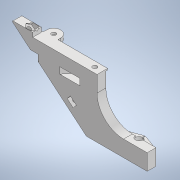
# Autodesk Inventor part: sciana
Saved by Autodesk Inventor 2022 (Build 260153000, 153)
## iProperties
Created: 2022-12-26
Part Number: sciana
Material: Generic
Document SubType Name: Modeling
Designer: Kamil
Density: 1 g/cm^3
Appearance: Default
Author: Kamil
Autodesk Inventor part; units mm, degrees
ref_plane "YZ Plane" through (0, 0, 0) normal (1, 0, 0) x (0, 1, 0)
ref_plane "XZ Plane" through (0, 0, 0) normal (0, 1, 0) x (-1, 0, 0)
ref_plane "XY Plane" through (0, 0, 0) normal (0, 0, 1) x (1, 0, 0)
sketch "Sketch1" plane through (0, 0, 0) normal (0, 0, 1) x (1, 0, 0)
  line L0 (7.1699, 8.5) -> (10.7451, 5.5) projected
  line L1 (65.8, 5.5) -> (10.7451, 5.5) projected
  line L2 (65.8, 5.5) -> (65.8, 8.5) projected
  line L3 (65.8, 8.5) -> (7.1699, 8.5) projected
  line L4 (10.7451, 5.5) -> (39.9536, -19.0089)
  circle A0 centre (83.9, -5.5) radius 16.1 projected
  line L5 (83.9, 8.5) -> (65.8, 8.5) projected
  line L6 (65.8, 5.5) -> (65.8, -20.8049)
  line L7 (65.8, -20.8049) -> (42.0941, -20.8049)
  line L8 (42.0941, -20.8049) -> (39.9536, -19.0089)
  circle A1 centre (83.9, -5.5) radius 18.1
  line L9 (83.9, -23.6) -> (100, -23.6)
  line L10 (100, -23.6) -> (100, -27.6)
  line L11 (100, -27.6) -> (50.1922, -27.6)
  line L12 (50.1922, -27.6) -> (42.0941, -20.8049)
  point P0 (0, 0)
  point P1 (65.8, -5.5)
  dimension "d0" = 4
  constraints: 16 end point, 3 perpendicular, 2 collinear, 2 horizontal, 2 vertical, 1 coincident, 3 other
  measures "d0" distance of L9.end L10.end
extrude "Extrusion1" add sketch "Sketch1" against normal blind 6 contours L1 L6 L7 L8 L4 | A1 L9 L10 L11 L12 L7 L6
sketch "Sketch2" plane through (10.7451, 5.5, 0) normal (0, 1, 0) x (1, 0, 0)
  line L0 (21.4448, 9) -> (21.4448, 14.7444) projected
  line L1 (85.3549, 52.5) -> (85.3549, 47.5) projected
  line L2 (85.3549, 47.5) -> (41.1549, 47.5) projected
  line L3 (41.1549, 47.5) -> (41.1549, 32) projected
  line L4 (41.1549, 32) -> (52.3217, 32) projected
  line L5 (52.3217, 32) -> (52.3217, 9) projected
  line L6 (52.3217, 9) -> (21.4448, 9) projected
  line L7 (21.4448, 9) -> (21.4448, 14.7444) projected
  line L8 (21.4448, 14.7444) -> (11.2254, 14.7444) projected
  line L9 (11.2254, 14.7444) -> (11.2254, 9) projected
  line L10 (11.2254, 9) -> (3.1975, 9) projected
  line L11 (3.1975, 9) -> (3.1975, 22) projected
  line L12 (3.1975, 22) -> (11.2254, 22) projected
  line L13 (11.2254, 22) -> (11.2254, 78) projected
  line L14 (11.2254, 78) -> (3.1975, 78) projected
  line L15 (3.1975, 78) -> (3.1975, 91) projected
  line L16 (3.1975, 91) -> (11.2254, 91) projected
  line L17 (11.2254, 91) -> (11.2254, 85.2556) projected
  line L18 (11.2254, 85.2556) -> (21.4448, 85.2556) projected
  line L19 (21.4448, 85.2556) -> (21.4448, 91) projected
  line L20 (21.4448, 91) -> (52.3217, 91) projected
  line L21 (52.3217, 91) -> (52.3217, 68) projected
  line L22 (52.3217, 68) -> (41.1549, 68) projected
  line L23 (41.1549, 68) -> (41.1549, 52.5) projected
  line L24 (41.1549, 52.5) -> (85.3549, 52.5) projected
  line L25 (22.6158, 64.3503) -> (20.3041, 53.9031) projected
  line L26 (20.3041, 53.9031) -> (21.8663, 53.5574) projected
  line L27 (21.8663, 53.5574) -> (24.178, 64.0047) projected
  line L28 (24.178, 64.0047) -> (22.6158, 64.3503) projected
  line L29 (20.2927, 51.2105) -> (22.6127, 40.765) projected
  line L30 (22.6127, 40.765) -> (24.1746, 41.112) projected
  line L31 (24.1746, 41.112) -> (21.8546, 51.5574) projected
  line L32 (21.8546, 51.5574) -> (20.2927, 51.2105) projected
  line L33 (25.3403, 18.5643) -> (24.1979, 17.4441) projected
  line L34 (24.1979, 17.4441) -> (31.6895, 9.8042) projected
  line L35 (31.6895, 9.8042) -> (32.8319, 10.9245) projected
  line L36 (32.8319, 10.9245) -> (25.3403, 18.5643) projected
  line L37 (37.3906, 88.6369) -> (36.265, 89.7739) projected
  line L38 (36.265, 89.7739) -> (28.6611, 82.2458) projected
  line L39 (28.6611, 82.2458) -> (29.7868, 81.1088) projected
  line L40 (29.7868, 81.1088) -> (37.3906, 88.6369) projected
  line L41 (37.3228, 15.3834) -> (36.9774, 13.8212) projected
  line L42 (36.9774, 13.8212) -> (47.4252, 11.5115) projected
  line L43 (47.4252, 11.5115) -> (47.7705, 13.0737) projected
  line L44 (47.7705, 13.0737) -> (37.3228, 15.3834) projected
  line L45 (51.9234, 89.2388) -> (51.5762, 90.8006) projected
  line L46 (51.5762, 90.8006) -> (41.1312, 88.4785) projected
  line L47 (41.1312, 88.4785) -> (41.4784, 86.9167) projected
  line L48 (41.4784, 86.9167) -> (51.9234, 89.2388) projected
  line L49 (39.447, 6) -> (0, 6) projected
  line L50 (0, 6) -> (55.0549, 6) projected
  line L51 (55.0549, 6) -> (73.1549, 6) projected
  line L52 (73.1549, 6) -> (89.2549, 6) projected
  line L53 (89.2549, 6) -> (39.447, 6) projected
  line L54 (16.3351, 14.7444) -> (16.3351, 5.7961)
  line L55 (39.447, 6) -> (0, 6) projected
  line L56 (16.3351, 6) -> (16.3351, 9.2)
  line L57 (14.4876, 6) -> (12.6401, 9.2)
  line L58 (12.6401, 9.2) -> (14.4876, 12.4)
  line L59 (14.4876, 12.4) -> (18.1826, 12.4)
  line L60 (18.1826, 12.4) -> (20.0302, 9.2)
  line L61 (20.0302, 9.2) -> (18.1826, 6)
  line L62 (18.1826, 6) -> (14.4876, 6)
  circle A0 centre (16.3351, 9.2) radius 4.75
  line L63 (11.5851, 9.2) -> (11.5851, 6)
  line L64 (21.0851, 9.2) -> (21.0851, 6)
  point P0 (-10.7451, 0)
  point P1 (11.5851, 6)
  point P2 (21.0851, 6)
  dimension "d3" = 3.2
  dimension "d4" = 9.5
  constraints: 20 end point, 5 point on line, 2 coincident, 2 midpoint, 2 perpendicular, 2 point on circle, 1 centre point, 1 tangent, 1 vertical, 13 other
  measures "d3" distance of L56.start L56.end
  measures "d4" diameter of A0
extrude "Extrusion2" add sketch "Sketch2" against normal blind 3 contours L61 L60 L59 L54 A0 L49 | A0 L64 L49 | L49 A0 L54 L59 L58 L57 | L49 L63 A0
sketch "Sketch3" plane through (10.7451, 5.5, 0) normal (0, 1, 0) x (1, 0, 0)
  line L0 (11.5851, 6) -> (14.4876, 6) projected
  line L1 (11.5851, 6) -> (11.5851, 9.2) projected
  arc A0 (21.0851, 9.2) -> (11.5851, 9.2) centre (16.3351, 9.2) ccw projected
  line L2 (21.0851, 9.2) -> (21.0851, 6) projected
  line L3 (18.1826, 6) -> (21.0851, 6) projected
  line L4 (18.1826, 6) -> (20.0302, 9.2) projected
  line L5 (20.0302, 9.2) -> (18.1826, 12.4) projected
  line L6 (18.1826, 12.4) -> (14.4876, 12.4) projected
  line L7 (14.4876, 12.4) -> (12.6401, 9.2) projected
  line L8 (12.6401, 9.2) -> (14.4876, 6) projected
  circle A1 centre (16.3351, 9.2) radius 1.5
  line L9 (14.4876, 6) -> (18.1826, 6) projected
  point P0 (-10.7451, 0)
  dimension "d7" = 3
  constraints: 1 centre point, 1 coincident
  measures "d7" diameter of A1
extrude "Extrusion3" add sketch "Sketch3" against normal blind 1.5 contours L8 L7 L6 L5 L4 L9
fillet "Fillet1" radius 2 4 edges at (31.8302, 4, -6) (22.3302, 4, -6) (30.379, 2.5, -6) (23.7815, 2.5, -6)
sketch "Sketch4" plane through (10.7451, 5.5, 0) normal (0, 1, 0) x (1, 0, 0)
  circle A0 centre (64.1549, 42.5) radius 1.75 projected
  circle A1 centre (64.1549, 57.5) radius 1.75 projected
  circle A2 centre (46.1549, 42.5) radius 1.5 projected
  circle A3 centre (46.1549, 57.5) radius 1.5 projected
  line L0 (-3.5753, 100) -> (-3.5753, 0) projected
  line L1 (55.0549, 0) -> (-3.5753, 0) projected
  line L2 (55.0549, 35) -> (55.0549, 0) projected
  line L3 (73.1549, 35) -> (55.0549, 35) projected
  line L4 (73.1549, 35) -> (73.1549, 65) projected
  line L5 (55.0549, 65) -> (73.1549, 65) projected
  line L6 (55.0549, 100) -> (55.0549, 65) projected
  line L7 (-3.5753, 100) -> (55.0549, 100) projected
  line L8 (23.0851, 6) -> (55.0549, 6) projected
  line L9 (55.0549, 0) -> (53.0549, 0)
  line L10 (53.0549, 0) -> (53.0549, 9.1684)
  line L11 (53.0549, 9.1684) -> (55.0549, 9.1684)
  line L12 (55.0549, 9.1684) -> (55.0549, 0)
  line L13 (53.0549, 0) -> (46.6549, 0)
  line L14 (46.6549, 0) -> (46.6549, 7.4)
  line L15 (46.6549, 7.4) -> (53.0549, 7.4)
  line L16 (53.0549, 7.4) -> (53.0549, 0)
  line L17 (46.6549, 3.7) -> (53.0549, 3.7)
  line L18 (46.6549, 5.5475) -> (49.8549, 7.395)
  line L19 (49.8549, 7.395) -> (53.0549, 5.5475)
  line L20 (53.0549, 5.5475) -> (53.0549, 1.8525)
  line L21 (53.0549, 1.8525) -> (49.8549, 0.005)
  line L22 (49.8549, 0.005) -> (46.6549, 1.8525)
  line L23 (46.6549, 1.8525) -> (46.6549, 5.5475)
  circle A4 centre (49.8549, 3.7) radius 1.5
  point P0 (-10.7451, 0)
  point P1 (46.6549, 1.8525)
  point P2 (53.0549, 1.8525)
  point P3 (53.0549, 6)
  point P4 (46.6549, 6)
  dimension "d11" = 2
  dimension "d12" = 6.4
  dimension "d13" = 7.4
  dimension "d14" = 3
  constraints: 30 end point, 4 midpoint, 4 parallel, 2 horizontal, 2 perpendicular, 1 centre point, 1 coincident, 13 other
  measures "d11" distance of L10.end L11.end
  measures "d12" distance of L14.end L15.end
  measures "d13" distance of L13.end L14.end
  measures "d14" diameter of A4
extrude "Extrusion4" cut sketch "Sketch4" against normal blind 10 contours L14 L17 A4 L10 L21 L22 | L14 L18 L8 L19 L10 L17 A4 | L14 L8 L18 | A4 L17 | L17 A4 | L10 L19 L8
sketch "Sketch5" plane through (10.7451, 5.5, 0) normal (0, 1, 0) x (1, 0, 0)
  line L0 (46.6549, 1.8525) -> (46.6549, 6) projected
  line L1 (23.0851, 6) -> (46.6549, 6) projected
  arc A0 (21.0851, 8) -> (23.0851, 6) centre (23.0851, 8) ccw projected
  line L2 (21.0851, 8) -> (21.0851, 9.2) projected
  arc A1 (21.0851, 9.2) -> (11.5851, 9.2) centre (16.3351, 9.2) ccw projected
  line L3 (11.5851, 9.2) -> (11.5851, 8) projected
  arc A2 (9.5851, 6) -> (11.5851, 8) centre (9.5851, 8) ccw projected
  line L4 (0, 6) -> (9.5851, 6) projected
  line L5 (0, 0) -> (0, 6) projected
  line L6 (55.0549, 0) -> (0, 0) projected
  line L7 (55.0549, 0) -> (55.0549, 6) projected
  line L8 (53.0549, 6) -> (55.0549, 6) projected
  line L9 (53.0549, 6) -> (53.0549, 1.8525) projected
  line L10 (53.0549, 1.8525) -> (49.8549, 0.005) projected
  line L11 (49.8549, 0.005) -> (46.6549, 1.8525) projected
  circle A3 centre (16.3351, 9.2) radius 1.5 projected
  line L12 (46.6549, 6) -> (53.0549, 6) projected
  line L13 (49.8549, 0.005) -> (49.8549, 7.405)
  line L14 (53.0549, 1.8525) -> (49.8549, 0.005) projected
  line L15 (49.8549, 0.005) -> (46.6506, 1.855)
  line L16 (46.6506, 1.855) -> (46.6506, 5.555)
  line L17 (46.6506, 5.555) -> (49.8549, 7.405)
  line L18 (49.8549, 7.405) -> (53.0592, 5.555)
  line L19 (53.0592, 5.555) -> (53.0592, 1.855)
  line L20 (53.0592, 1.855) -> (49.8549, 0.005)
  circle A4 centre (49.8549, 3.705) radius 1.5
  point P0 (-10.7451, 0)
  dimension "d17" = 7.4
  dimension "d18" = 3
  constraints: 14 end point, 2 point on line, 1 centre point, 1 coincident, 1 midpoint, 1 vertical, 13 other
  measures "d17" distance of L10.end L13.end
  measures "d18" diameter of A4
extrude "Extrusion5" add sketch "Sketch5" against normal blind 3 contours L0 L17 L12 L13 A4 L11 | L0 L12 L17 | L13 A4 L12 L18 L9 L10 | L18 L12 L9
extrude "Extrusion6" cut sketch "Sketch5" against normal through all contours A4 L13 | L13 A4
sketch "Sketch6" plane through (10.7451, -4.5, 0) normal (0, 1, 0) x (1, 0, 0)
  circle A0 centre (49.8549, 3.705) radius 1.5 projected
  line L0 (49.8549, 0.005) -> (46.6549, 1.8525) projected
  line L1 (53.0549, 1.8525) -> (49.8549, 0.005) projected
  line L2 (53.0549, 6) -> (53.0549, 1.8525) projected
  line L3 (46.6549, 6) -> (53.0549, 6) projected
  line L4 (46.6549, 1.8525) -> (46.6549, 6) projected
  line L5 (49.8549, 0.005) -> (46.6549, 1.8525) projected
  line L6 (49.427, 0.252) -> (50.2828, 0.252)
  line L7 (53.0549, 1.8525) -> (49.8549, 0.005) projected
  line L8 (46.6549, 6) -> (53.0549, 6) projected
  point P0 (-10.7451, 0)
  constraints: 2 end point, 2 point on line, 1 horizontal, 1 parallel
extrude "Extrusion7" add sketch "Sketch6" along normal up to surface (10 mm away) contours L0 L6 L1
sketch "Sketch7" plane through (10.7451, 5.5, 0) normal (0, 1, 0) x (1, 0, 0)
  circle A0 centre (49.8549, 3.705) radius 1.5 projected
  line L0 (23.0851, 6) -> (55.0549, 6) projected
  arc A1 (21.0851, 8) -> (23.0851, 6) centre (23.0851, 8) ccw projected
  line L1 (21.0851, 8) -> (21.0851, 9.2) projected
  arc A2 (21.0851, 9.2) -> (11.5851, 9.2) centre (16.3351, 9.2) ccw projected
  line L2 (11.5851, 9.2) -> (11.5851, 8) projected
  arc A3 (9.5851, 6) -> (11.5851, 8) centre (9.5851, 8) ccw projected
  line L3 (0, 6) -> (9.5851, 6) projected
  line L4 (0, 0) -> (0, 6) projected
  line L5 (55.0549, 0) -> (0, 0) projected
  line L6 (55.0549, 0) -> (55.0549, 6) projected
  circle A4 centre (16.3351, 9.2) radius 1.5 projected
  line L7 (23.0851, 6) -> (55.0549, 6) projected
  line L8 (55.0549, 6) -> (0, 6)
  line L9 (0, 6) -> (0, 7.2)
  line L10 (0, 7.2) -> (55.0549, 7.2)
  line L11 (55.0549, 7.2) -> (55.0549, 6)
  arc A5 (21.0851, 8) -> (23.0851, 6) centre (23.0851, 8) ccw projected
  line L12 (21.2521, 7.2) -> (21.2521, 6)
  line L13 (39.447, 6) -> (0, 6) projected
  point P0 (-10.7451, 0)
  point P1 (21.2521, 7.2)
  dimension "d25" = 1.2
  constraints: 10 end point, 2 parallel, 2 perpendicular, 2 point on line, 1 horizontal, 1 point on circle
  measures "d25" distance of L8.end L9.end
extrude "Extrusion8" add sketch "Sketch7" against normal blind 1 contours A1 L10 L11 L0
sketch "Sketch8" plane through (50.1922, -27.6, 0) normal (0, -1, 0) x (1, 0, 0)
  circle A0 centre (10.4078, -3.705) radius 1.5 projected
  line L0 (0, 0) -> (49.8078, 0) projected
  line L1 (0, 0) -> (0, -6) projected
  line L2 (49.8078, -6) -> (0, -6) projected
  line L3 (49.8078, 0) -> (49.8078, -6) projected
  point P0 (-50.1922, 0)
extrude "Extrusion9" add sketch "Sketch8" along normal blind 7 contours A0 | L0 L3 L2 L1
sketch "Sketch9" plane through (83.9, -23.6, 0) normal (0, 1, 0) x (1, 0, 0)
  line L0 (2.04, 37.5) -> (2.04, 35) projected
  line L1 (2.04, 35) -> (7.04, 35) projected
  line L2 (7.04, 35) -> (7.04, 37.5) projected
  arc A0 (7.04, 37.5) -> (2.04, 37.5) centre (4.54, 37.5) ccw projected
  line L3 (2.04, 65) -> (2.04, 62.5) projected
  arc A1 (2.04, 62.5) -> (7.04, 62.5) centre (4.54, 62.5) ccw projected
  line L4 (7.04, 62.5) -> (7.04, 65) projected
  line L5 (7.04, 65) -> (2.04, 65) projected
  line L6 (-34.4121, 91) -> (12.2, 91) projected
  line L7 (12.2, 91) -> (12.2, 9) projected
  line L8 (12.2, 9) -> (-34.4121, 9) projected
  line L9 (-34.4121, 9) -> (-34.4121, 35.1398) projected
  line L10 (-34.4121, 35.1398) -> (-18.3552, 35.1398) projected
  line L11 (-18.3552, 35.1398) -> (2.6186, 47.1223) projected
  line L12 (2.6186, 47.1223) -> (2.6186, 52.8777) projected
  line L13 (2.6186, 52.8777) -> (-18.6, 65) projected
  line L14 (-18.6, 65) -> (-34.4121, 65) projected
  line L15 (-34.4121, 65) -> (-34.4121, 91) projected
  circle A2 centre (9, 57.5) radius 1.75 projected
  circle A3 centre (9, 42.5) radius 1.75 projected
  line L16 (-33.7078, 6) -> (16.1, 6) projected
  line L17 (16.1, 6) -> (16.1, 0) projected
  line L18 (16.1, 0) -> (-33.7078, 0) projected
  line L19 (-33.7078, 0) -> (-33.7078, 6) projected
  line L20 (7.04, 35) -> (2.04, 35)
  line L21 (2.04, 35) -> (2.04, -1.5182)
  line L22 (2.04, -1.5182) -> (7.04, -1.5182)
  line L23 (7.04, -1.5182) -> (7.04, 35)
  line L24 (0, 6) -> (16.1, 6) projected
  line L25 (7.04, 6) -> (2.04, 6)
  circle A4 centre (4.54, 6) radius 4
  circle A5 centre (4.54, 6) radius 2.5
  line L26 (16.1, 6) -> (5.9241, 9.7529)
  line L27 (-33.7078, 6) -> (16.1, 6) projected
  line L28 (5.9241, 9.7529) -> (3.156, 9.7529)
  line L29 (4.54, 6) -> (4.54, 7.154)
  line L30 (-7.0199, 6) -> (3.156, 9.7529)
  point P0 (-83.9, 0)
  point P1 (7.04, 6)
  point P2 (-7.0199, 6)
  dimension "d30" = 8
  dimension "d31" = 5
  constraints: 18 end point, 4 point on line, 2 centre point, 2 horizontal, 2 parallel, 2 point on circle, 1 coincident, 1 midpoint, 1 perpendicular, 1 symmetric about line, 1 tangent, 1 vertical
  measures "d30" diameter of A4
  measures "d31" diameter of A5
extrude "Extrusion10" add sketch "Sketch9" against normal blind 4 contours L30 A4 L21 | L21 A4 L8 L30 | L26 L8 A4 L23 | L23 A4 L26 | A4 L28 L23 L8 L21 | L21 L8 A4 | L8 A4 L16 L30 | A4 L28 | A4 L8 L23 | L26 L16 A4 L8 | L21 L16 A4 L8 | L8 L23 A5 L21 | L8 A4 L16 L23
sketch "Sketch10" plane through (83.9, -23.6, 0) normal (0, 1, 0) x (1, 0, 0)
  line L0 (0, 0) -> (0, 6) projected
  line L1 (16.1, 0) -> (0, 0) projected
  line L2 (16.1, 0) -> (16.1, 6) projected
  line L3 (16.1, 6) -> (5.9241, 9.7529) projected
  arc A0 (5.9241, 9.7529) -> (3.156, 9.7529) centre (4.54, 6) ccw projected
  line L4 (3.156, 9.7529) -> (-7.0199, 6) projected
  line L5 (0, 6) -> (-7.0199, 6) projected
  arc A1 (7.04, 6) -> (2.04, 6) centre (4.54, 6) ccw projected
  line L6 (2.04, 6) -> (7.04, 6) projected
  line L7 (-33.7078, 6) -> (16.1, 6) projected
  line L8 (-7.0199, 6) -> (16.1, 6)
  line L9 (4.54, 8.5) -> (4.54, 10)
  line L10 (4.54, 10) -> (4.24, 10)
  line L11 (4.24, 10) -> (4.24, 7.3138)
  line L12 (4.24, 7.3138) -> (4.54, 7.3138)
  line L13 (4.54, 7.3138) -> (4.54, 10)
  line L14 (4.24, 10) -> (4.84, 10)
  line L15 (4.84, 10) -> (4.84, 7.3138)
  line L16 (4.84, 7.3138) -> (4.24, 7.3138)
  line L17 (4.24, 7.3138) -> (4.24, 10)
  line L18 (4.84, 10) -> (4.24, 10)
  line L19 (4.24, 10) -> (4.24, 10.5275)
  line L20 (4.24, 10.5275) -> (4.84, 10.5275)
  line L21 (4.84, 10.5275) -> (4.84, 10)
  point P0 (-83.9, 0)
  point P1 (4.24, 10)
  dimension "d34" = 0.3
  dimension "d35" = 0.6
  constraints: 28 end point, 6 parallel, 4 horizontal, 3 perpendicular, 2 point on circle, 2 point on line
  measures "d34" distance of L12.end L11.end
  measures "d35" distance of L15.end L16.end
extrude "Extrusion11" cut sketch "Sketch10" against normal blind 1 contours L5 L4 A0 L11 A1 L7 | L7 A1 L15 A0 L3 | L11 A0 L9 A1 | L9 A0 L15 A1
extrude "Extrusion12" cut sketch "Sketch10" against normal blind 2 contours L11 A0 L9 A1 | A1 L13 L12 L11 | L11 L10 A0 | L9 A0 L15 A1 | A1 L15 L16 L13 | A0 L14 L15 | L10 L19 L20 L21 L14
sketch "Sketch11" plane through (83.9, -23.6, 0) normal (0, 1, 0) x (1, 0, 0)
  line L0 (0, 6) -> (16.1, 6) projected
  line L1 (0, 0) -> (0, 6) projected
  line L2 (16.1, 0) -> (0, 0) projected
  line L3 (16.1, 0) -> (16.1, 6) projected
  line L4 (4.84, 9.9887) -> (4.84, 8.4819) projected
  arc A0 (7.04, 6) -> (4.84, 8.4819) centre (4.54, 6) ccw projected
  line L5 (16.1, 6) -> (7.04, 6) projected
  line L6 (5.9241, 9.7529) -> (16.1, 6) projected
  arc A1 (5.9241, 9.7529) -> (4.84, 9.9887) centre (4.54, 6) ccw projected
  line L7 (4.24, 8.4819) -> (4.24, 9.9887) projected
  arc A2 (4.24, 9.9887) -> (3.156, 9.7529) centre (4.54, 6) ccw projected
  line L8 (-7.0199, 6) -> (3.156, 9.7529) projected
  line L9 (2.04, 6) -> (-7.0199, 6) projected
  arc A3 (4.24, 8.4819) -> (2.04, 6) centre (4.54, 6) ccw projected
  arc A4 (4.84, 8.4819) -> (4.24, 8.4819) centre (4.54, 6) ccw projected
  circle A5 centre (4.54, 6) radius 2.5
  point P0 (-83.9, 0)
  constraints: 1 centre point, 1 coincident
extrude "Extrusion13" cut sketch "Sketch11" against normal through all contours L0 A5
sketch "Sketch12" plane through (0, 0, 0) normal (0, 0, 1) x (1, 0, 0)
  line L0 (10.7451, 5.5) -> (50.1922, -27.6) projected
  line L1 (50.1922, -27.6) -> (50.1922, -34.6) projected
  line L2 (100, -34.6) -> (50.1922, -34.6) projected
  line L3 (100, -34.6) -> (100, -23.6) projected
  line L4 (100, -23.6) -> (83.9, -23.6) projected
  arc A0 (65.8, -5.5) -> (83.9, -23.6) centre (83.9, -5.5) ccw projected
  line L5 (65.8, -5.5) -> (65.8, 5.5) projected
  line L6 (65.8, 5.5) -> (10.7451, 5.5) projected
  line L7 (50.1922, -27.6) -> (71.1014, -45.1449)
  line L8 (10.7451, 5.5) -> (50.1922, -27.6) projected
  point P0 (0, 0)
  point P1 (50.1922, -27.6)
  point P2 (58.5344, -34.6)
  constraints: 2 end point, 1 collinear
extrude "Extrusion14" cut sketch "Sketch12" against normal blind 10 contours L7 L2 L1
ref_plane "Work Plane1" through (31.9898, -6.0133, 20.6968) normal (0, -1, 0) x (0, 0, 1)
sketch "Sketch13" plane through (31.9898, -6.0133, 20.6968) normal (0, -1, 0) x (0, 0, 1)
  line L0 (-33.0166, -25.0895) -> (35.0823, -6.204)
  line L1 (19.121, 25.0895) -> (-35.0823, -21.2045)
  line L2 (-35.0823, -21.2045) -> (-33.0166, -25.0895)
  line L3 (35.0823, -6.204) -> (19.121, 25.0895)
  line L4 (-20.6968, -26.5446) -> (-26.6968, -26.5446) projected
  line L5 (-26.6968, -26.5446) -> (-26.6968, -53.9502) projected
  arc A0 (-26.6968, -58.9502) -> (-26.6968, -53.9502) centre (-26.6968, -56.4502) ccw projected
  line L6 (-26.6968, -58.9502) -> (-26.6968, -68.0102) projected
  line L7 (-26.6968, -68.0102) -> (-20.6968, -68.0102) projected
  line L8 (-20.6968, -68.0102) -> (-20.6968, -26.5446) projected
  point P0 (-20.6968, 31.9898)
  constraints: 8 end point, 8 other
ref_plane "Work Plane2" through (6.9003, -3.6133, -14.3854) normal (0, 1, 0) x (0, 0, 1)
extrude "Extrusion15" cut sketch "Sketch13" against normal up to surface (2.4 mm away) contours L2 L1 L3 L0
ref_plane "Work Plane3" through (8.1777, -6.0133, 8.6215) normal (0, -1, 0) x (0, 0, 1)
sketch "Sketch14" plane through (8.1777, -6.0133, 8.6215) normal (0, -1, 0) x (0, 0, 1)
  line L0 (3.0626, 38.2053) -> (-26.1922, -24.5344)
  line L1 (-22.0032, -27.7487) -> (35.8312, 20.7819)
  line L2 (35.8312, 20.7819) -> (3.0626, 38.2053)
  line L3 (-26.1922, -24.5344) -> (-22.0032, -27.7487)
  line L4 (-20.7347, -49.2901) -> (60.9839, -26.6275)
  line L5 (41.8304, 10.9246) -> (-23.2135, -44.6281)
  line L6 (-23.2135, -44.6281) -> (-20.7347, -49.2901)
  line L7 (60.9839, -26.6275) -> (41.8304, 10.9246)
  point P0 (-8.6215, 8.1777)
  point P1 (-24.0977, -26.1415)
  point P2 (-21.9741, -46.9591)
  constraints: 16 end point
extrude "Extrusion16" cut sketch "Sketch14" against normal blind 3.4
extrude "Extrusion17" cut sketch "Sketch14" along normal blind 1
sketch "Sketch15" plane through (10.7451, 5.5, -6) normal (-0.6427876, -0.7660444, 0) x (0.7660444, -0.6427876, 0)
  circle A0 centre (4.0467, 3) radius 1.5
  point P0 (-4.6959, 6)
  constraints: 1 centre point, 2 other
extrude "Extrusion18" cut sketch "Sketch15" against normal blind 5
sketch "Sketch16" plane through (10.7451, 5.5, -6) normal (-0.6427876, -0.7660444, 0) x (0.7660444, -0.6427876, 0)
  line L0 (12.622, 6) -> (-7.9342, 6)
  line L1 (12.622, 0) -> (0, 0) projected
  circle A0 centre (4.0467, 3) radius 1.5
  line L2 (0, 6) -> (0, 0) projected
  line L3 (12.622, 6) -> (12.622, -5.8362)
  line L4 (42.1745, 6) -> (0, 6) projected
  line L5 (10.5566, 0) -> (7.3426, 0) projected
  line L6 (0, 6) -> (7.8944, 6)
  line L7 (7.8944, 6) -> (7.8944, 0)
  line L8 (7.8944, 0) -> (0, 0)
  line L9 (0, 0) -> (0, 6)
  point P0 (-4.6959, 6)
  constraints: 12 end point, 2 horizontal, 2 parallel, 1 centre point, 1 perpendicular, 1 point on line, 1 vertical, 5 other
extrude "Extrusion19" cut sketch "Sketch16" against normal blind 7 contours L7 L1 L2 L0
extrude "Extrusion20" add sketch "Sketch16" against normal blind 7 contours L7 L1 L2 L0
sketch "Sketch17" plane through (15.2446, 10.8623, -6) normal (0.6427876, 0.7660444, 0) x (0.7660444, -0.6427876, 0)
  line L0 (0, -6) -> (7.8944, -6) projected
  line L1 (7.8944, -6) -> (7.8944, 0) projected
  line L2 (7.8944, 0) -> (0, 0) projected
  line L3 (0, 0) -> (0, -6) projected
  circle A0 centre (4.0467, -3) radius 1.5 projected
  line L4 (4.0467, -3) -> (6.7967, -3)
  line L5 (4.0467, -3) -> (4.0467, -5.75)
  circle A1 centre (4.0467, -3) radius 1.5 projected
  line L6 (2.459, -5.75) -> (0.8713, -3)
  line L7 (0.8713, -3) -> (2.459, -0.25)
  line L8 (2.459, -0.25) -> (5.6345, -0.25)
  line L9 (5.6345, -0.25) -> (7.2222, -3)
  line L10 (7.2222, -3) -> (5.6345, -5.75)
  line L11 (5.6345, -5.75) -> (2.459, -5.75)
  point P0 (-4.6959, -6)
  dimension "d56" = 2.75
  dimension "d57" = 2.75
  constraints: 16 end point, 1 coincident, 1 horizontal, 1 midpoint, 1 vertical, 13 other
  measures "d56" distance of L4.start L4.end
  measures "d57" distance of L4.start L5.end
extrude "Extrusion21" cut sketch "Sketch17" against normal blind 3 contours L6 L7 L8 L9 L10 L11
extrude "Extrusion22" add sketch "Sketch17" along normal blind 3 contours L3 L2 L1 L0
sketch "Sketch18" plane through (0, 0, 0) normal (0, 0, 1) x (1, 0, 0)
  line L0 (23.5488, 8.5) -> (23.5488, 5.5)
  line L1 (66.2988, 8.5) -> (23.1699, 8.5)
  line L2 (7.1699, 8.5) -> (23.1699, 8.5)
  line L3 (10.7451, 5.5) -> (20.4141, -2.6133) projected
  line L4 (20.4141, -2.6133) -> (24.6974, -2.6133) projected
  line L5 (24.6974, -2.6133) -> (24.6974, -6.2073) projected
  line L6 (24.6974, -6.2073) -> (58.5344, -34.6) projected
  line L7 (100, -34.6) -> (58.5344, -34.6) projected
  line L8 (100, -34.6) -> (100, -23.6) projected
  line L9 (100, -23.6) -> (83.9, -23.6) projected
  arc A0 (65.8, -5.5) -> (83.9, -23.6) centre (83.9, -5.5) ccw projected
  line L10 (65.8, -5.5) -> (65.8, 5.5) projected
  line L11 (65.8, 5.5) -> (21.0505, 5.5) projected
  line L12 (21.0505, 5.5) -> (23.2205, 8.086) projected
  line L13 (17.173, 13.1604) -> (23.2205, 8.086) projected
  line L14 (10.7451, 5.5) -> (17.173, 13.1604) projected
  line L15 (54.1085, -2.6133) -> (54.1085, -7.0133) projected
  line L16 (54.1085, -7.0133) -> (40.3431, -7.0133) projected
  line L17 (40.3431, -7.0133) -> (40.3431, -2.6133) projected
  line L18 (40.3431, -2.6133) -> (54.1085, -2.6133) projected
  line L19 (-2.1895, 16.3535) -> (63.3263, -38.6208)
  point P0 (0, 0)
  point P1 (22.7271, 8.5)
  point P2 (13.2624, 8.5)
  constraints: 8 end point, 2 horizontal, 1 vertical, 8 other
extrude "Extrusion23" add sketch "Sketch18" against normal up to surface (6 mm away) contours L0 L11 L12 L13 L2 L1 | L14 L19 L2
extrude "Extrusion24" cut sketch "Sketch18" against normal through all contours L2 L14 L13
sketch "Sketch19" plane through (7.1699, 8.5, 0) normal (0, 1, 0) x (1, 0, 0)
  line L0 (15.5204, 3) -> (13.4478, 5.75) projected
  line L1 (13.4478, 0.25) -> (15.5204, 3) projected
  line L2 (9.3026, 0.25) -> (13.4478, 0.25) projected
  line L3 (7.23, 3) -> (9.3026, 0.25) projected
  line L4 (9.3026, 5.75) -> (7.23, 3) projected
  line L5 (13.4478, 5.75) -> (9.3026, 5.75) projected
  line L6 (0, 6) -> (16.3789, 6) projected
  line L7 (0, 0) -> (0, 6) projected
  line L8 (16.3789, 0) -> (0, 0) projected
  line L9 (16.3789, 0) -> (16.3789, 6) projected
  line L10 (16.3789, 0) -> (16.3789, 6) projected
  line L11 (13.1604, 6) -> (16.3789, 6) projected
  line L12 (16.3789, 0) -> (14.7697, 0)
  line L13 (14.7697, 0) -> (14.7697, 6)
  line L14 (14.7697, 6) -> (16.3789, 6)
  line L15 (16.3789, 6) -> (16.3789, 0)
  point P0 (-7.1699, 0)
  constraints: 8 end point, 2 parallel, 1 horizontal, 1 midpoint, 1 perpendicular
extrude "Extrusion25" cut sketch "Sketch19" against normal up to surface (3 mm away) contours L1 L13 L0 | L0 L13 L6 L9 L8 L1
sketch "Sketch20" plane through (10.7451, 4, 0) normal (0, -1, 0) x (1, 0, 0)
  line L0 (20.0302, -9.2) -> (18.1826, -12.4) projected
  line L1 (18.1826, -6) -> (20.0302, -9.2) projected
  line L2 (14.4876, -6) -> (18.1826, -6) projected
  line L3 (12.6401, -9.2) -> (14.4876, -6) projected
  line L4 (14.4876, -12.4) -> (12.6401, -9.2) projected
  line L5 (18.1826, -12.4) -> (14.4876, -12.4) projected
  circle A0 centre (16.3351, -9.2) radius 1.5 projected
  line L6 (16.3351, -9.2) -> (16.3351, -6.45)
  line L7 (17.9228, -6.45) -> (19.5105, -9.2)
  line L8 (19.5105, -9.2) -> (17.9228, -11.95)
  line L9 (17.9228, -11.95) -> (14.7474, -11.95)
  line L10 (14.7474, -11.95) -> (13.1597, -9.2)
  line L11 (13.1597, -9.2) -> (14.7474, -6.45)
  line L12 (14.7474, -6.45) -> (17.9228, -6.45)
  point P0 (-10.7451, 0)
  point P1 (16.3351, -9.2)
  dimension "d68" = 2.75
  constraints: 14 end point, 1 midpoint, 1 vertical, 13 other
  measures "d68" distance of L6.start L6.end
extrude "Extrusion26" add sketch "Sketch20" along normal blind 4 contours L0 L5 L4 L3 L2 L1
sketch "Sketch21" plane through (22.3302, 2.5, -9.2) normal (-1, 0, 0) x (0, 0, 1)
  line L0 (0, 0) -> (1.2, 0) projected
  line L1 (0, 0) -> (0, -2.5) projected
  line L2 (3.2, -2.5) -> (0, -2.5) projected
  line L3 (3.2, -2) -> (3.2, -2.5) projected
  arc A0 (3.2, -2) -> (1.2, 0) centre (1.2, -2) ccw projected
  line L4 (-3.2, 0) -> (0, 0) projected
  line L5 (-3.2, 0) -> (-3.2, -2.5) projected
  line L6 (0, -2.5) -> (-3.2, -2.5) projected
  line L7 (0, 0) -> (0, -2.5) projected
  point P0 (9.2, -2.5)
extrude "Extrusion27" cut sketch "Sketch21" against normal through all
sketch "Sketch22" plane through (10.7451, 2.5, 0) normal (0, -1, 0) x (1, 0, 0)
  circle A0 centre (49.8549, -3.705) radius 1.5 projected
  line L0 (50.2828, -0.252) -> (49.427, -0.252) projected
  line L1 (46.6549, -1.8525) -> (49.427, -0.252) projected
  line L2 (46.6549, -6) -> (46.6549, -1.8525) projected
  line L3 (46.6549, -6) -> (53.0549, -6) projected
  line L4 (53.0549, -1.8525) -> (53.0549, -6) projected
  line L5 (50.2828, -0.252) -> (53.0549, -1.8525) projected
  line L6 (49.8549, -3.705) -> (47.1049, -3.705)
  line L7 (55.0549, 0) -> (11.1944, 0) projected
  line L8 (47.1049, -2.1172) -> (49.8549, -0.5295)
  line L9 (49.8549, -0.5295) -> (52.6049, -2.1172)
  line L10 (52.6049, -2.1172) -> (52.6049, -5.2927)
  line L11 (52.6049, -5.2927) -> (49.8549, -6.8804)
  line L12 (49.8549, -6.8804) -> (47.1049, -5.2927)
  line L13 (47.1049, -5.2927) -> (47.1049, -2.1172)
  line L14 (47.1049, -5.2927) -> (47.1049, -6)
  line L15 (52.6049, -5.2661) -> (52.6049, -6)
  point P0 (-10.7451, 0)
  point P1 (52.6049, -5.2927)
  dimension "d73" = 2.75
  constraints: 18 end point, 3 point on line, 2 vertical, 1 coincident, 1 midpoint, 1 parallel, 13 other
  measures "d73" distance of L6.start L6.end
extrude "Extrusion28" add sketch "Sketch22" along normal blind 10 contours L5 L4 L3 L15 L10 L9 L8 L13 L14 L2 L1 L0
fillet "Fillet2" radius 0.5 2 edges at (24.6974, -4.4103, 0) (7.1699, 8.5, -3)
sketch "Sketch24" plane through (58.5344, -34.6, -6) normal (-0.6427876, -0.7660444, 0) x (0.7660444, -0.6427876, 0)
  circle A0 centre (-17.5598, 2.5) radius 1.5
  line L0 (-17.5598, 2.5) -> (-14.8098, 2.5)
  ellipse E0 centre (-42.7714, 5.5) end of major axis (-43.4241, 5.5) minor radius 0.5 (-42.7714, 6) -> (-43.2714, 5.1786) ccw projected
  line L1 (-43.2714, 5.1786) -> (-42.9173, 4.8554) projected
  line L2 (-42.9173, 4.8554) -> (-42.9173, 0) projected
  line L3 (0, 0) -> (-42.9173, 0) projected
  line L4 (0, 6) -> (0, 0) projected
  line L5 (-42.7714, 6) -> (0, 6) projected
  line L6 (-14.8098, 0.9123) -> (-17.5598, -0.6754)
  line L7 (-17.5598, -0.6754) -> (-20.3098, 0.9123)
  line L8 (-20.3098, 0.9123) -> (-20.3098, 4.0877)
  line L9 (-20.3098, 4.0877) -> (-17.5598, 5.6754)
  line L10 (-17.5598, 5.6754) -> (-14.8098, 4.0877)
  line L11 (-14.8098, 4.0877) -> (-14.8098, 0.9123)
  line L12 (-14.8098, 4.0877) -> (-14.8098, 6.5068)
  line L13 (-14.8098, 6.5068) -> (-20.3098, 6.5068)
  line L14 (-20.3098, 4.0877) -> (-20.3098, 6.5068)
  line L15 (-20.21, 6) -> (-20.21, -1.2) projected
  point P0 (-67.0804, 6)
  point P1 (-14.8098, 6)
  point P2 (-20.21, 0.8547)
  point P3 (-18.7297, 0)
  point P4 (-16.3899, 0)
  dimension "d79" = 2.75
  constraints: 20 end point, 2 parallel, 2 perpendicular, 1 centre point, 1 coincident, 1 midpoint, 16 other
  measures "d79" distance of L0.start L0.end
extrude "Extrusion30" cut sketch "Sketch24" against normal blind 7 contours A0 | L5 L12 L10 L9 L15 | L9 L10 L11 L6 L3 L7 L15
extrude "Extrusion31" add sketch "Sketch24" against normal blind 3.6 contours L5 L12 L10 L9 L15 | L9 L10 L11 L6 L3 L7 L15
sketch "Sketch25" plane through (58.5344, -34.6, -6) normal (-0.6427876, -0.7660444, 0) x (0.7660444, -0.6427876, 0)
  circle A0 centre (-17.5598, 2.5) radius 1.5
  point P0 (-67.0804, 6)
  constraints: 1 centre point, 2 other
extrude "Extrusion32" cut sketch "Sketch25" against normal blind 13
body "Solid1"
